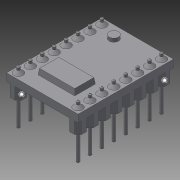
# Autodesk Inventor part: DRV8825_Pololu_Carrier
Saved by Autodesk Inventor 2014 (Build 180170000, 170)
## iProperties
Created: 2014-11-10
Part Number: DRV8825_Pololu_Carrier
Material: Generic
Document SubType Name: Modeling
Designer: ThatOtherGuy
Density: 1 g/cm^3
Appearance: Default
Author: ThatOtherGuy
Autodesk Inventor part; units mm, degrees
ref_plane "YZ Plane" through (0, 0, 0) normal (1, 0, 0) x (0, 1, 0)
ref_plane "XZ Plane" through (0, 0, 0) normal (0, 1, 0) x (-1, 0, 0)
ref_plane "XY Plane" through (0, 0, 0) normal (0, 0, 1) x (1, 0, 0)
sketch "Sketch1" plane through (0, 0, 0) normal (0, 0, 1) x (1, 0, 0)
  line L0 (0, 0) -> (15.24, 0)
  line L1 (15.24, 0) -> (15.24, 20.32)
  line L2 (15.24, 20.32) -> (0, 20.32)
  line L3 (0, 20.32) -> (0, 0)
  dimension "d0" = 15.24
  dimension "d1" = 20.32
  constraints: 8 end point, 2 parallel, 1 horizontal, 1 perpendicular
  measures "d0" distance of L1.end L2.end
  measures "d1" distance of L2.end L0.start
extrude "Board" add sketch "Sketch1" along normal blind 1.6
sketch "Sketch4" plane through (0, 0, 0) normal (0, 0, -1) x (-1, 0, 0)
  line L0 (0, 0) -> (-15.24, 0) projected
  line L1 (0, 20.32) -> (0, 0) projected
  line L2 (-1.7961, 2.54) -> (-0.7439, 2.54)
  line L3 (-0.7439, 2.54) -> (0, 1.7961)
  line L4 (0, 1.7961) -> (0, 0.7439)
  line L5 (0, 0.7439) -> (-0.7439, 0)
  line L6 (-0.7439, 0) -> (-1.7961, 0)
  line L7 (-1.7961, 0) -> (-2.54, 0.7439)
  line L8 (-2.54, 0.7439) -> (-2.54, 1.7961)
  line L9 (-2.54, 1.7961) -> (-1.7961, 2.54)
  point P0 (-1.27, 1.27)
  dimension "d24" = 2.54
  dimension "d25" = 1.27
  dimension "d26" = 1.27
  constraints: 16 end point, 1 horizontal, 17 other
  measures "d24" distance between parallel lines of L6 L2
  measures "d25" distance from line of L0 point (-1.27, 1.27)
  measures "d26" distance from line of L1 point (-1.27, 1.27)
extrude "Bottom_Header" add sketch "Sketch4" along normal blind 2.54 contours L0 L7 L8 L9 L2 L3 L1 L5
sketch "Sketch5" plane through (0, 0, -2.54) normal (0, 0, -1) x (-1, 0, 0)
  line L0 (-0.7439, 2.54) -> (-1.7961, 2.54) projected
  line L1 (-2.54, 1.7961) -> (-2.54, 0.7439) projected
  circle A0 centre (-1.27, 1.27) radius 0.325
  point P0 (0, 0)
  point P1 (-2.54, 1.27)
  point P2 (-1.27, 2.54)
  dimension "d35" = 0.65
  constraints: 2 midpoint, 1 centre point, 1 horizontal alignment, 1 vertical alignment
  measures "d35" diameter of A0
extrude "Bottom_Pin" add sketch "Sketch5" along normal blind 6
fillet "Bottom_Pin_Point" radius 0.1905 1 edges at (1.595, 1.27, -8.54)
pattern_linear "Bottom_Headers" count 8 spacing 2.54 along (0, 1, 0) count 2 spacing 12.7 along (1, 0, 0) of "Bottom_Header", "Bottom_Pin", "Bottom_Pin_Point"
sketch "Sketch3" plane through (0, 0, 1.6) normal (0, 0, 1) x (1, 0, 0)
  circle A0 centre (1.27, 1.27) radius 0.325
  point P0 (0, 0)
  dimension "d9" = 0.65
  dimension "d10" = 1.27
  dimension "d11" = 1.27
  constraints: 1 centre point
  measures "d9" diameter of A0
  measures "d10" horizontal distance of point (0, 0) A0.centre
  measures "d11" horizontal distance of point (0, 0) A0.centre
extrude "Top_Pin" add sketch "Sketch3" along normal blind 1.27
fillet "Top_Pin_Point" radius 0.1905 1 edges at (0.945, 1.27, 2.87)
chamfer "Top_Pin_Solder" distance 0.635 angle 45 1 edges at (0.945, 1.27, 1.6)
pattern_linear "Top_Pins" count 8 spacing 2.54 along (0, 1, 0) count 2 spacing 12.7 along (1, 0, 0) of "Top_Pin", "Top_Pin_Point", "Top_Pin_Solder"
sketch "Sketch6" plane through (0, 0, 1.6) normal (0, 0, 1) x (1, 0, 0)
  line L0 (0, 0) -> (15.24, 0) projected
  line L1 (15.24, 20.32) -> (0, 20.32) projected
  line L2 (3.72, 7.4) -> (11.52, 7.4)
  line L3 (11.52, 7.4) -> (11.52, 3)
  line L4 (11.52, 3) -> (3.72, 3)
  line L5 (3.72, 3) -> (3.72, 7.4)
  point P0 (7.62, 7.4)
  point P1 (7.62, 20.32)
  dimension "d39" = 7.8
  dimension "d40" = 3
  dimension "d41" = 4.4
  constraints: 8 end point, 2 midpoint, 2 parallel, 1 horizontal, 1 perpendicular, 1 vertical alignment
  measures "d39" distance of L2.start L2.end
  measures "d40" distance between parallel lines of L4 L0
  measures "d41" distance of L4.end L2.start
extrude "DRV8825" add sketch "Sketch6" along normal blind 1.2 draft -7.5
sketch "Sketch7" plane through (0, 0, 1.6) normal (0, 0, 1) x (1, 0, 0)
  line L0 (15.24, 20.32) -> (0, 20.32) projected
  line L1 (0, 20.32) -> (0, 0) projected
  circle A0 centre (5.08, 17.78) radius 1
  dimension "d44" = 2.54
  dimension "d45" = 5.08
  dimension "d46" = 2
  constraints: 1 centre point
  measures "d44" distance from line of L0 A0.centre
  measures "d45" distance from line of L1 A0.centre
  measures "d46" diameter of A0
extrude "DRV8825_Pot" add sketch "Sketch7" along normal blind 0.75
equation "\"d25\" = 0.5 * d24"
equation "\"d26\" = d25"
body "Solid1"
